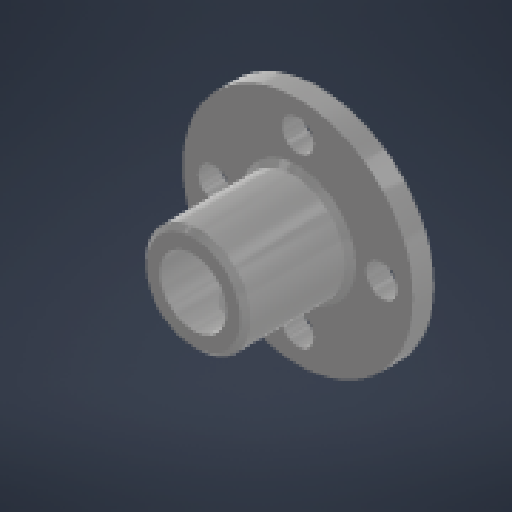
# Autodesk Inventor part: mặt bích
Saved by Autodesk Inventor 2027.1 (Build 311270010, 270A)
## iProperties
Created: 2026-06-14
Part Number: mặt bích
Material: Generic
Document SubType Name: Sheet Metal
Designer: MSI
Density: 1 g/cm^3
Sheet Metal Rule: Default_mm
Appearance: Smooth - Medium Gray
Author: MSI
Autodesk Inventor part; units mm, degrees
ref_plane "YZ Plane" through (0, 0, 0) normal (1, 0, 0) x (0, 1, 0)
ref_plane "XZ Plane" through (0, 0, 0) normal (0, 1, 0) x (-1, 0, 0)
ref_plane "XY Plane" through (0, 0, 0) normal (0, 0, 1) x (1, 0, 0)
sketch "Sketch1" plane through (0, 0, 0) normal (0, 0, 1) x (1, 0, 0)
  circle A0 centre (0, 0) radius 3.175
  circle A1 centre (0, 0) radius 5
  circle A2 centre (0, 0) radius 11
  circle A3 centre (0, 8) radius 1.5
  circle A4 centre (-8, 0) radius 1.5
  circle A5 centre (0, -8) radius 1.5
  circle A6 centre (8, 0) radius 1.5
  dimension "d0" = 22
  dimension "d1" = 6.35
  dimension "d2" = 10
  dimension "d3" = 3
  dimension "d4" = 8
  dimension "d7" = 360
  constraints: 8 coincident, 7 centre point, 15 other
  measures "d0" diameter of A2
  measures "d1" diameter of A0
  measures "d2" diameter of A1
  measures "d3" diameter of A3
  measures "d4" distance of A3.centre point (0, 0)
extrude "Extrusion1" add sketch "Sketch1" along normal blind 12 contours A1
extrude "Extrusion2" add sketch "Sketch1" along normal blind 2 contours A2
chamfer "Chamfer1" distance 0.5 angle 45 2 edges at (-5, 0, 2) (-5, 0, 12)
sketch "Sketch3" plane through (0, 0, 0) normal (0, 1, 0) x (-1, 0, 0)
  circle A0 centre (0, 7.5211) radius 1.5
  point P0 (0, 0)
  dimension "d16" = 3
  constraints: 1 centre point
  measures "d16" diameter of A0
extrude "Extrusion3" cut sketch "Sketch3" against normal blind 10
equation "\"BendRadius\" = Thickness"
equation "\"BendReliefWidth\" = Thickness"
equation "\"BendReliefDepth\" = 0.5 * Thickness"
equation "\"CornerReliefSize\" = 4 * Thickness"
equation "\"MinimumRemnant\" = 2 * Thickness"
equation "\"TransitionRadius\" = BendRadius"
equation "\"JacobiRadiusSize\" = BendRadius"
equation "\"GapSize\" = Thickness"
equation "\"Thickness\" = 0.5"
body "Solid1"
